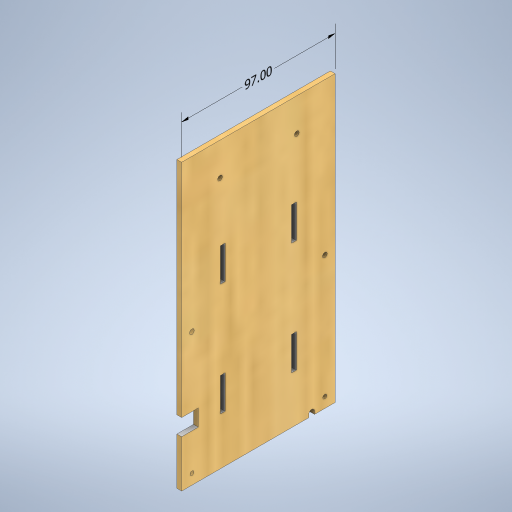
# Autodesk Inventor part: Panel2
Saved by Autodesk Inventor 2023 (Build 270158000, 158)
## iProperties
Created: 2022-12-03
Part Number: Panel2
Material: Genérico
Document SubType Name: Modeling
Designer: sergi
Density: 1 g/cm^3
Appearance: Valor por defecto
Author: sergi
Autodesk Inventor part; units mm, degrees
ref_plane "YZ Plane" through (0, 0, 0) normal (1, 0, 0) x (0, 1, 0)
ref_plane "XZ Plane" through (0, 0, 0) normal (0, 1, 0) x (-1, 0, 0)
ref_plane "XY Plane" through (0, 0, 0) normal (0, 0, 1) x (1, 0, 0)
sketch "Boceto1" plane through (0, 0, 0) normal (0, 1, 0) x (-1, 0, 0)
  line L0 (-1.5, -48.5) -> (1.5, -48.5)
  line L1 (1.5, -48.5) -> (1.5, 48.5)
  line L2 (1.5, 48.5) -> (-1.5, 48.5)
  line L3 (-1.5, 48.5) -> (-1.5, -48.5)
  line L4 (-1.5, -48.5) -> (1.5, 48.5) construction
  line L5 (1.5, -48.5) -> (-1.5, 48.5) construction
  point P0 (0, 0)
  dimension "d0" = 3
  dimension "d1" = 97
  constraints: 12 end point, 2 midpoint, 2 parallel, 1 horizontal, 1 perpendicular
  measures "d0" distance of L2.end L1.end
  measures "d1" distance of L1.end L0.end
extrude "Extrusión1" add sketch "Boceto1" along normal blind 180
sketch "Boceto2" plane through (-1.5, 0, -48.5) normal (-1, 0, 0) x (0, 0, 1)
  circle A0 centre (24.25, 159.25) radius 1.5 projected
  circle A1 centre (72.75, 159.25) radius 1.5 projected
  circle A2 centre (90.5, 84) radius 1.5 projected
  circle A3 centre (6.5, 84) radius 1.5 projected
  circle A4 centre (6.5, 6.5) radius 1.25 projected
  circle A5 centre (90.5, 6.5) radius 1.25 projected
  point P0 (48.5, 0)
extrude "Extrusión2" cut sketch "Boceto2" against normal through all
sketch "Boceto3" plane through (1.5, 0, 48.5) normal (1, 0, 0) x (0, 0, -1)
  line L0 (10.5, 26) -> (5.5, 26)
  line L1 (10.5, 44) -> (10.5, 26)
  line L2 (5.5, 44) -> (-0.0781, 44)
  line L3 (-0.0781, 26) -> (5.5, 26)
  line L4 (0, 0) -> (0, 180) projected
  line L5 (0, 44) -> (10.5, 44)
  line L6 (10.5, 44) -> (10.5, 26)
  line L7 (10.5, 26) -> (0, 26)
  line L8 (0, 26) -> (0, 44)
  line L9 (0, 35) -> (10.5, 35)
  line L10 (10.5, 29.75) -> (0, 29.75)
  line L11 (0, 29.75) -> (0, 40.25)
  line L12 (0, 40.25) -> (10.5, 40.25)
  line L13 (10.5, 40.25) -> (10.5, 29.75)
  line L14 (10.5, 29.75) -> (0, 40.25) construction
  line L15 (0, 29.75) -> (10.5, 40.25) construction
  point P0 (48.5, 0)
  point P1 (5.25, 35)
  point P2 (10.5, 40.25)
  point P3 (10.5, 29.75)
  dimension "d13" = 10.5
  constraints: 30 end point, 5 midpoint, 5 parallel, 4 horizontal, 3 point on line, 2 perpendicular
  measures "d13" distance of L10.end L11.end
extrude "Extrusión3" cut sketch "Boceto3" against normal through all contours L10 L4 L9 L1 | L9 L4 L12 L1
sketch "Boceto4" plane through (1.5, 0, 48.5) normal (1, 0, 0) x (0, 0, -1)
  line L0 (84, 0) -> (84, 13) projected
  line L1 (100, 0) -> (-3, 0) projected
  arc A0 (84, 1.85) -> (80.3, 1.85) centre (82.15, 1.85) ccw
  line L2 (0, 0) -> (97, 0) projected
  line L3 (80.3, 1.85) -> (80.3, 0)
  line L4 (97, 0) -> (0, 0) projected
  line L5 (84, 1.85) -> (84, 0)
  point P0 (48.5, 0)
  dimension "d9" = 3.7
  constraints: 4 end point, 3 tangent, 2 point on circle, 2 point on line, 1 centre point, 1 collinear, 1 perpendicular
  measures "d9" diameter of A0
extrude "Extrusión4" cut sketch "Boceto4" against normal through all
sketch "Boceto5" plane through (1.5, 0, -48.5) normal (1, 0, 0) x (0, 0, -1)
  line L0 (-48.5, 0) -> (-72.5, 0)
  line L1 (-16.7, 0) -> (-97, 0) projected
  line L2 (-72.5, 0) -> (-72.5, 30)
  line L3 (-97, 0) -> (-16.7, 0) projected
  line L4 (-72.5, 30) -> (-69.5, 30)
  line L5 (-69.5, 30) -> (-69.5, 51)
  line L6 (-69.5, 51) -> (-72.5, 51)
  line L7 (-72.5, 51) -> (-72.5, 30)
  line L8 (-48.5, 0) -> (-24.5, 0)
  line L9 (-24.5, 0) -> (-24.5, 30)
  line L10 (-24.5, 30) -> (-27.5, 30)
  line L11 (-27.5, 30) -> (-27.5, 51.0089)
  line L12 (-27.5, 51.0089) -> (-24.5, 51.0089)
  line L13 (-24.5, 51.0089) -> (-24.5, 30)
  line L14 (-72.5, 51) -> (-72.5, 101)
  line L15 (-72.5, 101) -> (-69.5, 101)
  line L16 (-69.5, 101) -> (-69.5, 122)
  line L17 (-69.5, 122) -> (-72.5, 122)
  line L18 (-72.5, 122) -> (-72.5, 101)
  line L19 (-27.5, 101) -> (-24.5, 101)
  line L20 (-24.5, 101) -> (-24.5, 122)
  line L21 (-24.5, 122) -> (-27.5, 122)
  line L22 (-27.5, 122) -> (-27.5, 101)
  dimension "d14" = 24
  dimension "d15" = 30
  dimension "d16" = 3
  dimension "d17" = 21
  dimension "d18" = 24
  dimension "d19" = 30
  dimension "d20" = 3
  dimension "d21" = 50
  dimension "d22" = 21
  constraints: 42 end point, 14 perpendicular, 9 point on line, 1 collinear, 1 horizontal, 1 vertical
  measures "d14" distance of L0.start L0.end
  measures "d15" distance of L0.end L2.end
  measures "d16" distance of L2.end L4.end
  measures "d17" distance of L4.end L5.end
  measures "d18" distance of L0.start L8.end
  measures "d19" distance of L8.end L9.end
  measures "d20" distance of L9.end L10.end
  measures "d21" distance of L6.end L14.end
  measures "d22" distance of L15.end L16.end
extrude "Extrusión5" cut sketch "Boceto5" against normal blind 10
